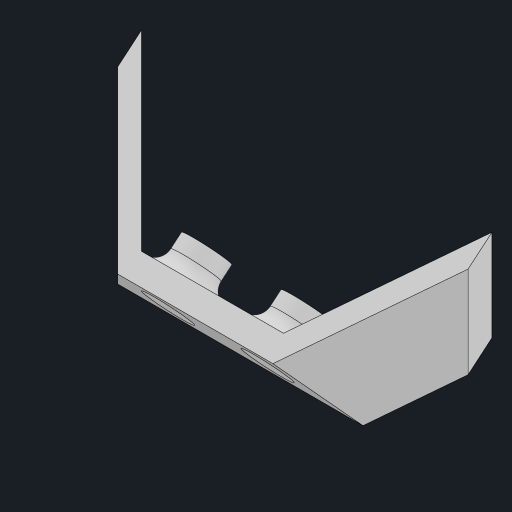
# Autodesk Inventor part: om_Drop_bumper
Saved by Autodesk Inventor 2023 (Build 270158000, 158)
## iProperties
Created: 2022-06-21
Part Number: om_Drop_bumper
Material: 一般
Document SubType Name: Modeling
Designer: legot
Density: 1 g/cm^3
Appearance: 既定
Author: legot
Autodesk Inventor part; units mm, degrees
ref_plane "YZ Plane" through (0, 0, 0) normal (1, 0, 0) x (0, 1, 0)
ref_plane "XZ Plane" through (0, 0, 0) normal (0, 1, 0) x (-1, 0, 0)
ref_plane "XY Plane" through (0, 0, 0) normal (0, 0, 1) x (1, 0, 0)
sketch "スケッチ1" plane through (0, 0, 0) normal (0, 1, 0) x (-1, 0, 0)
  line L0 (28.2843, -28.2843) -> (0, 0)
  line L1 (0, 0) -> (-28.2843, -28.2843)
  line L2 (29.9813, -26.5872) -> (0, 3.3941)
  line L3 (0, 3.3941) -> (-29.9813, -26.5872)
  line L4 (28.2843, -28.2843) -> (29.9813, -26.5872)
  line L5 (-28.2843, -28.2843) -> (-29.9813, -26.5872)
  dimension "d0" = 40
  dimension "d1" = 2.4
  constraints: 13 end point, 5 perpendicular, 1 horizontal alignment, 1 other
  measures "d0" distance of L0.start L0.end
  measures "d1" distance of L0.start L2.start
extrude "押し出し1" add sketch "スケッチ1" along normal blind 50
sketch "スケッチ2" plane through (0, 0, 0) normal (1, 0, 0) x (0, 1, 0)
  line L0 (0, 3.3941) -> (31.9749, -34.7121)
  line L1 (0, 0) -> (0, -28.2843) projected
  line L2 (7.6604, 9.822) -> (39.6354, -28.2843)
  line L3 (0, 3.3941) -> (7.6604, 9.822)
  line L4 (39.6354, -28.2843) -> (31.9749, -34.7121)
  line L5 (0, -28.2843) -> (50, -28.2843) projected
  point P0 (26.5813, -28.2843)
  dimension "d4" = 40
  dimension "d5" = 10
  constraints: 9 end point, 2 perpendicular, 1 parallel, 1 point on line
  measures "d4" angle of L0 L1
  measures "d5" distance between parallel lines of L2 L0
extrude "押し出し2" cut sketch "スケッチ2" along normal mid plane 50 contours L3 L2 L5 L0 keep common part
ref_plane "作業平面1" through (0, 9.2239, 0.1802) normal (0, 0.7660444, 0.6427876) x (0.7938448, -0.3908923, 0.4658473)
sketch "スケッチ4" plane through (0, 9.2239, 0.1802) normal (0, 0.7660444, 0.6427876) x (0.7938448, -0.3908923, 0.4658473)
  line L0 (-37.1409, 7.3737) -> (2.5514, 37.7797)
  line L1 (-34.5895, 4.0431) -> (-39.6922, 10.7043) projected
  line L2 (0, 41.1103) -> (5.1027, 34.4491) projected
  point P0 (3.5216, -4.5971)
  constraints: 2 end point, 2 midpoint
ref_plane "作業平面2" through (-25, 27.5045, -21.6059) normal (0, -0.6427876, 0.7660444) x (1, 0, 0)
sketch "スケッチ6" plane through (0, 9.2239, 0.1802) normal (0, 0.7660444, 0.6427876) x (0.7938448, -0.3908923, 0.4658473)
  line L0 (5.1027, -6.6611) -> (-34.5895, 4.0431) projected
  line L1 (5.1027, 34.4491) -> (5.1027, -6.6611) projected
  line L2 (5.1027, -6.6611) -> (-22.6818, 0.8318)
  line L3 (-22.6818, 0.8318) -> (5.1027, 22.116)
  line L4 (5.1027, 22.116) -> (5.1027, -6.6611)
  point P0 (3.5216, -4.5971)
  point P1 (5.1027, 22.116)
  dimension "d17" = 35
  constraints: 6 end point, 2 collinear, 1 equal length
  measures "d17" distance of L2.end L3.end
extrude "押し出し3" cut sketch "スケッチ6" along normal mid plane 50
sketch "スケッチ7" plane through (14.1059, 14.6842, -14.1059) normal (0, -0.6427876, 0.7660444) x (1, 0, 0)
  line L0 (3.3941, 0) -> (0, 0) projected
  line L1 (-3.0338, 10) -> (3.3941, 0) projected
  line L2 (-6.4279, 10) -> (-3.0338, 10) projected
  line L3 (-31.6059, 0) -> (-25.178, 10) projected
  line L4 (-28.2118, 0) -> (-31.6059, 0) projected
  line L5 (-21.7839, 10) -> (-28.2118, 0) projected
  line L6 (-25.178, 10) -> (-21.7839, 10) projected
  line L7 (-21.7839, 10) -> (-6.4279, 10)
  line L8 (-28.2118, 0) -> (0, 0)
  point P0 (-14.1059, -2.1817)
  constraints: 4 end point
extrude "押し出し4" add sketch "スケッチ7" against normal blind 3.2
sketch "スケッチ5" plane through (-25, 27.5045, -21.6059) normal (0, -0.6427876, 0.7660444) x (1, 0, 0)
  line L0 (0, 0) -> (50, 0) projected
  line L1 (17.9, 0) -> (32.1, 0)
  point P0 (25, -7.1817)
  point P1 (25, 0)
  dimension "d9" = 14.2
  constraints: 2 end point, 2 midpoint, 2 point on line, 1 collinear
  measures "d9" distance of L1.start L1.end
hole "穴1" at (-7.1, 27.5045, -21.6059) at (7.1, 27.5045, -21.6059) direction (0, -0.6427876, 0.7660444) diameter 4 end through all
sketch "スケッチ9" plane through (14.1059, 16.7412, -16.5572) normal (0, 0.6427876, -0.7660444) x (-1, 0, 0)
  circle A0 centre (21.2059, 5) radius 2 construction
  circle A1 centre (7.0059, 5) radius 2 construction
  circle A2 centre (7.0059, 5) radius 1.25
  circle A3 centre (7.0059, 5) radius 3
  circle A4 centre (21.2059, 5) radius 1.25
  circle A5 centre (21.2059, 5) radius 3
  point P0 (14.1059, -2.1817)
  dimension "d22" = 2.5
  dimension "d23" = 1
  constraints: 4 centre point, 2 equal radius
  measures "d22" diameter of A2
  measures "d23" radial gap between concentric circles of A1 A3
extrude "押し出し5" add sketch "スケッチ9" along normal blind 4
fillet "フィレット1" radius 2 2 edges at (-4.1, 20.5714, -13.3433) (10.1, 20.5714, -13.3433)
chamfer "面取り1" distance 1.2 angle 45 2 edges at (7.1, 16.9824, -12.1775) (-7.1, 16.9824, -12.1775)
